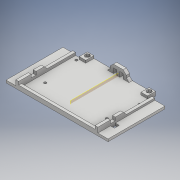
# Autodesk Inventor part: odroid_router
Saved by Autodesk Inventor 2018 (Build 220112000, 112)
## iProperties
Created: 2018-05-15
Part Number: odroid_router
Material: Generic
Document SubType Name: Modeling
Designer: bitbots
Density: 1 g/cm^3
Appearance: Default
Author: bitbots
Autodesk Inventor part; units mm, degrees
ref_plane "YZ Plane" through (0, 0, 0) normal (1, 0, 0) x (0, 1, 0)
ref_plane "XZ Plane" through (0, 0, 0) normal (0, 1, 0) x (-1, 0, 0)
ref_plane "Work Plane1" through (0, 0, 2) normal (0, 0, 1) x (1, 0, 0)
sketch "Sketch1" plane through (0, 0, 2) normal (0, 0, 1) x (1, 0, 0)
  arc A0 (0, 3.5) -> (-3.5, 0) centre (0, 0) ccw construction
  line L0 (-3.5, -52) -> (-3.5, 0) construction
  arc A1 (-3.5, -52) -> (0, -55.5) centre (0, -52) ccw construction
  line L1 (76, -55.5) -> (0, -55.5) construction
  arc A2 (76, -55.5) -> (79.5, -52) centre (76, -52) ccw construction
  line L2 (79.5, 0) -> (79.5, -52) construction
  arc A3 (79.5, 0) -> (76, 3.5) centre (76, 0) ccw construction
  line L3 (0, 3.5) -> (76, 3.5) construction
  circle A4 centre (0, -52) radius 1.4224 construction
  circle A5 centre (0, 0) radius 1.4224 construction
  circle A6 centre (76, 0) radius 1.4224 construction
  circle A7 centre (76, -52) radius 1.4224 construction
  circle A8 centre (25.43, -38.5) radius 1.4224 construction
  circle A9 centre (76.11, -18.5) radius 1.4224 construction
  circle A10 centre (76, 0) radius 1.5
  circle A11 centre (76, -52) radius 1.5
  circle A12 centre (76, -52) radius 3.5
  circle A13 centre (76, 0) radius 3.5
  circle A14 centre (0, -52) radius 1.5
  circle A15 centre (0, -52) radius 3.5
  circle A16 centre (0, 0) radius 1.5
  circle A17 centre (0, 0) radius 3.5
  dimension "d0" = 3
  dimension "d1" = 3
  dimension "d2" = 7
  dimension "d3" = 7
  dimension "d4" = 3
  dimension "d5" = 7
  dimension "d6" = 3
  dimension "d7" = 7
  constraints: 8 centre point, 8 coincident
  measures "d0" diameter of A10
  measures "d1" diameter of A11
  measures "d2" diameter of A12
  measures "d3" diameter of A13
  measures "d4" diameter of A14
  measures "d5" diameter of A15
  measures "d6" diameter of A16
  measures "d7" diameter of A17
extrude "Extrusion1" add sketch "Sketch1" against normal blind 4.5
sketch "Sketch2" plane through (0, 0, 2) normal (0, 0, 1) x (1, 0, 0)
  circle A0 centre (76, -52) radius 1.5 projected
  circle A1 centre (76, -52) radius 3.5 projected
  circle A2 centre (0, -52) radius 3.5 projected
  circle A3 centre (0, 0) radius 1.5 projected
  circle A4 centre (0, 0) radius 3.5 projected
  circle A5 centre (76, 0) radius 1.5 projected
  circle A6 centre (76, 0) radius 3.5 projected
  circle A7 centre (76, -52) radius 1.5 projected
  line L0 (76, -52) -> (76, -56)
  circle A8 centre (76, -52) radius 3.5 projected
  circle A9 centre (0, 0) radius 3.5 projected
  line L1 (0, 0) -> (-4, 0)
  circle A10 centre (0, -52) radius 1.5 projected
  circle A11 centre (0, -52) radius 3.5 projected
  line L2 (76, -56) -> (80, -56)
  line L3 (-4, 0) -> (-4, 4)
  line L4 (-4, 4) -> (80, 4)
  line L5 (80, 4) -> (80, -56)
  line L6 (80, -56) -> (-4, -56)
  line L7 (-4, -56) -> (-4, 4)
  point P0 (0, 0)
  dimension "d10" = 4
  dimension "d12" = 4
  dimension "d21" = 4
  dimension "d22" = 4
  constraints: 16 end point, 3 horizontal, 2 parallel, 2 vertical, 1 perpendicular, 1 vertical alignment
  measures "d10" distance of L0.start L0.end
  measures "d12" distance of L1.start L1.end
  measures "d21" distance of L0.end L2.end
  measures "d22" distance of L1.end L3.end
extrude "Extrusion2" add sketch "Sketch2" along normal blind 2 contours A1 | A4 | L6 L7 L3 L4 L5 L2 | A2 | A6
sketch "Sketch3" plane through (0, 0, 4) normal (0, 0, 1) x (1, 0, 0)
  circle A0 centre (76, 0) radius 1.5 construction
  circle A1 centre (0, 0) radius 1.5 construction
  circle A2 centre (0, -52) radius 1.5 construction
  circle A3 centre (76, -52) radius 1.5 construction
  circle A4 centre (0, 0) radius 1.5 construction
  line L0 (0, 0) -> (2.6, 0) construction
  line L1 (2.6, -1.5011) -> (0, -3.0022)
  line L2 (0, -3.0022) -> (-2.6, -1.5011)
  line L3 (-2.6, -1.5011) -> (-2.6, 1.5011)
  line L4 (-2.6, 1.5011) -> (0, 3.0022)
  line L5 (0, 3.0022) -> (2.6, 1.5011)
  line L6 (2.6, 1.5011) -> (2.6, -1.5011)
  line L7 (3.3236, -3.218) -> (-3.3236, 3.218) construction
  line L8 (-3.3236, -3.218) -> (3.3236, 3.218) construction
  line L9 (80, 4) -> (-4, 4) projected
  line L10 (-4, 4) -> (-4, -56) projected
  line L11 (4, -4) -> (-4, -4)
  line L12 (-4, -4) -> (-4, 4)
  line L13 (-4, 4) -> (4, 4)
  line L14 (4, 4) -> (4, -4)
  circle A5 centre (0, 0) radius 1.5 projected
  line L15 (4, -4) -> (-4, 4) construction
  line L16 (-4, -4) -> (4, 4) construction
  point P0 (0, 0)
  dimension "d18" = 2.6
  constraints: 30 end point, 5 midpoint, 2 horizontal, 2 parallel, 1 coincident, 1 perpendicular, 13 other
  measures "d18" distance of L0.start L0.end
extrude "Extrusion3" add sketch "Sketch3" along normal blind 3 contours L14 L11 L10 L9
ref_plane "Work Plane2" through (38, -56, 2) normal (1, 0, 0) x (0, 0, -1)
mirror "Mirror1" about plane through (38, -56, 2) normal (1, 0, 0) of "Extrusion3"
sketch "Sketch4" plane through (0, 0, 4) normal (0, 0, 1) x (1, 0, 0)
  circle A0 centre (76, -52) radius 1.5 projected
  circle A1 centre (0, -52) radius 1.5 projected
  line L0 (80, -4) -> (72, -4) projected
  line L1 (72, -4) -> (72, 4) projected
  line L2 (72, 4) -> (4, 4) projected
  line L3 (4, 4) -> (4, -4) projected
  line L4 (4, -4) -> (-4, -4) projected
  line L5 (-4, -4) -> (-4, -56) projected
  line L6 (-4, -56) -> (80, -56) projected
  line L7 (80, -56) -> (80, -4) projected
  line L8 (-4, 4) -> (-4, -56) projected
  line L9 (-4, -56) -> (-4, 4)
  line L10 (-4, -26) -> (38, -26)
  line L11 (-11, -48) -> (87, -48)
  line L12 (87, -48) -> (87, -4)
  line L13 (87, -4) -> (-11, -4)
  line L14 (-11, -4) -> (-11, -48)
  line L15 (-11, -48) -> (87, -4) construction
  line L16 (87, -48) -> (-11, -4) construction
  point P0 (0, 0)
  dimension "d23" = 98
  dimension "d24" = 44
  constraints: 16 end point, 3 midpoint, 2 horizontal, 2 parallel, 1 perpendicular, 1 vertical
  measures "d23" distance of L13.end L12.end
  measures "d24" distance of L11.end L12.end
extrude "Extrusion4" add sketch "Sketch4" against normal blind 2 contours L7 L11 L5 L4 L13 L0 | L13 L12 L11 L7 | L11 L14 L13 L5
sketch "Sketch5" plane through (0, 0, 4) normal (0, 0, 1) x (1, 0, 0)
  circle A0 centre (76, 0) radius 1.5 projected
  line L0 (76, 0) -> (76, -20)
  line L1 (76, -20) -> (81, -20)
  circle A1 centre (81, -20) radius 1.5
  circle A2 centre (0, 0) radius 1.5 projected
  line L2 (0, 0) -> (0, -12)
  line L3 (0, -12) -> (-5, -12)
  circle A3 centre (-5, -12) radius 1.5
  point P0 (0, 0)
  dimension "d27" = 20
  dimension "d28" = 5
  dimension "d29" = 3
  dimension "d30" = 12
  dimension "d31" = 5
  dimension "d32" = 3
  constraints: 8 end point, 2 centre point, 2 coincident, 2 vertical, 1 horizontal, 1 perpendicular
  measures "d27" distance of L0.start L0.end
  measures "d28" distance of L0.end L1.end
  measures "d29" diameter of A1
  measures "d30" distance of L2.start L2.end
  measures "d31" distance of L2.end L3.end
  measures "d32" diameter of A3
extrude "Extrusion5" cut sketch "Sketch5" against normal blind 2 contours A1 | A3
sketch "Sketch7" plane through (-11, -48, 4) normal (-1, 0, 0) x (0, 0, 1)
  line L0 (0, 44) -> (0, 0) projected
  line L1 (0, 44) -> (-2, 44) projected
  line L2 (-2, 0) -> (-2, 44) projected
  line L3 (0, 0) -> (-2, 0) projected
  point P0 (-4, 48)
extrude "Extrusion6" add sketch "Sketch7" along normal blind 3
sketch "Sketch6" plane through (0, 0, 4) normal (0, 0, 1) x (1, 0, 0)
  circle A0 centre (81, -20) radius 1.5 projected
  circle A1 centre (-5, -12) radius 1.5 projected
  circle A2 centre (0, -52) radius 1.5 projected
  circle A3 centre (76, -52) radius 1.5 projected
  line L0 (72, -4) -> (72, 4) projected
  line L1 (72, 4) -> (4, 4) projected
  line L2 (4, 4) -> (4, -4) projected
  line L3 (4, -4) -> (-4, -4) projected
  line L4 (-4, -4) -> (-14, -4) projected
  line L5 (-14, -48) -> (-4, -48) projected
  line L6 (-4, -48) -> (-4, -56) projected
  line L7 (-4, -56) -> (80, -56) projected
  line L8 (80, -56) -> (80, -48) projected
  line L9 (80, -48) -> (87, -48) projected
  line L10 (87, -48) -> (87, -4) projected
  line L11 (87, -4) -> (80, -4) projected
  line L12 (80, -4) -> (72, -4) projected
  line L13 (81, -20) -> (83.5, -20)
  line L14 (83.5, -20) -> (83.5, -4)
  line L15 (80, -4) -> (87, -4) projected
  line L16 (87, -4) -> (83.5, -4)
  line L17 (87, -48) -> (87, -4) projected
  line L18 (87, -4) -> (87, -48)
  line L19 (83.5, -20) -> (83.5, -48)
  line L20 (80, -48) -> (87, -48) projected
  line L21 (87, -48) -> (83.5, -48)
  circle A4 centre (-5, -12) radius 1.5 projected
  line L22 (-5, -12) -> (-10.5, -12)
  line L23 (-14, -48) -> (-14, -4) projected
  line L24 (-10.5, -12) -> (-10.5, -4)
  line L25 (-4, -4) -> (-14, -4) projected
  line L26 (-14, -4) -> (-10.5, -4)
  line L27 (-4, -48) -> (-14, -48) projected
  line L28 (-14, -4) -> (-14, -48)
  line L29 (-14, -48) -> (-10.5, -48)
  line L30 (-10.5, -48) -> (-10.5, -12)
  point P0 (0, 0)
  dimension "d35" = 2.5
  dimension "d36" = 5.5
  constraints: 24 end point, 5 collinear, 3 point on line, 2 horizontal, 2 midpoint, 2 vertical
  measures "d35" distance of L13.start L13.end
  measures "d36" distance of L22.start L22.end
extrude "Extrusion7" add sketch "Sketch6" along normal blind 3.3 contours L14 L11 L10 L9 L19 | L5 L23 L4 L24 L30
sketch "Sketch8" plane through (0, 0, 4) normal (0, 0, 1) x (1, 0, 0)
  line L0 (83.5, -48) -> (83.5, -4) projected
  line L1 (83.5, -4) -> (80, -4) projected
  line L2 (80, -4) -> (72, -4) projected
  line L3 (72, -4) -> (72, 4) projected
  line L4 (72, 4) -> (4, 4) projected
  line L5 (4, 4) -> (4, -4) projected
  line L6 (4, -4) -> (-4, -4) projected
  line L7 (-4, -4) -> (-10.5, -4) projected
  line L8 (-10.5, -4) -> (-10.5, -48) projected
  line L9 (-10.5, -48) -> (-4, -48) projected
  line L10 (-4, -48) -> (-4, -56) projected
  line L11 (-4, -56) -> (80, -56) projected
  line L12 (80, -56) -> (80, -48) projected
  line L13 (80, -48) -> (83.5, -48) projected
  circle A0 centre (81, -20) radius 1.5 projected
  circle A1 centre (-5, -12) radius 1.5 projected
  circle A2 centre (0, -52) radius 1.5 projected
  circle A3 centre (76, -52) radius 1.5 projected
  circle A4 centre (81, -20) radius 1.5 projected
  line L14 (81, -20) -> (81, -74)
  line L15 (-14, -4) -> (-14, -48) projected
  line L16 (-14, -48) -> (-10.5, -48) projected
  line L17 (-10.5, -48) -> (-10.5, -4) projected
  line L18 (-10.5, -4) -> (-14, -4) projected
  line L19 (87, -48) -> (87, -4) projected
  line L20 (87, -4) -> (83.5, -4) projected
  line L21 (83.5, -4) -> (83.5, -48) projected
  line L22 (83.5, -48) -> (87, -48) projected
  line L23 (81, -74) -> (87, -74)
  line L24 (80, -48) -> (87, -48)
  line L25 (87, -48) -> (87, -74)
  line L26 (87, -74) -> (80, -74)
  line L27 (80, -74) -> (80, -48)
  line L28 (-10.5, -48) -> (-4, -48)
  line L29 (-4, -48) -> (-4, -74)
  line L30 (-4, -74) -> (-10.5, -74)
  line L31 (-10.5, -74) -> (-10.5, -48)
  line L32 (-4, -74) -> (80, -74)
  line L33 (80, -74) -> (80, -56)
  line L34 (80, -56) -> (-4, -56)
  line L35 (-4, -56) -> (-4, -74)
  line L36 (-4, -48) -> (-14, -48) projected
  line L37 (-14, -48) -> (-10.5, -48)
  line L38 (-10.5, -48) -> (-10.5, -74)
  line L39 (-10.5, -74) -> (-14, -74)
  line L40 (-14, -74) -> (-14, -48)
  point P0 (0, 0)
  dimension "d41" = 54
  constraints: 36 end point, 8 parallel, 5 horizontal, 4 perpendicular, 1 point on line, 1 vertical
  measures "d41" distance of L14.start L14.end
extrude "Extrusion8" add sketch "Sketch8" against normal blind 2 contours L22 L25 L23 L14 L13 | L14 L26 L27 L12 L13 | L27 L32 L29 L11 | L29 L30 L31 L9 L10 | L39 L40 L16 L31 | L16 L15 L18 L8
sketch "Sketch9" plane through (0, 0, 4) normal (0, 0, 1) x (1, 0, 0)
  line L0 (83.5, -48) -> (83.5, -4) projected
  line L1 (83.5, -4) -> (80, -4) construction
  line L2 (80, -4) -> (72, -4) construction
  line L3 (72, -4) -> (72, 4) construction
  line L4 (72, 4) -> (4, 4) construction
  line L5 (4, 4) -> (4, -4) construction
  line L6 (4, -4) -> (-4, -4) construction
  line L7 (-4, -4) -> (-10.5, -4) projected
  line L8 (-10.5, -4) -> (-10.5, -48) projected
  line L9 (-14, -48) -> (-10.5, -48) projected
  line L10 (-14, -48) -> (-14, -74) projected
  line L11 (-14, -74) -> (87, -74) projected
  line L12 (87, -74) -> (87, -48) projected
  line L13 (83.5, -48) -> (87, -48) projected
  circle A0 centre (81, -20) radius 1.5 construction
  circle A1 centre (-5, -12) radius 1.5 projected
  circle A2 centre (0, -52) radius 1.5 projected
  circle A3 centre (76, -52) radius 1.5 projected
  line L14 (-14, -74) -> (87, -74) projected
  line L15 (-14, -48) -> (-10.5, -48)
  line L16 (-10.5, -48) -> (-10.5, -74)
  line L17 (-10.5, -74) -> (-14, -74)
  line L18 (-14, -74) -> (-14, -48)
  line L19 (87, -48) -> (87, -4) projected
  line L20 (87, -48) -> (83.5, -48)
  line L21 (83.5, -48) -> (83.5, -74)
  line L22 (83.5, -74) -> (87, -74)
  line L23 (87, -74) -> (87, -48)
  line L24 (83.5, -74) -> (-10.5, -74)
  line L25 (-10.5, -74) -> (-10.5, -70.7)
  line L26 (-10.5, -70.7) -> (83.5, -70.7)
  line L27 (83.5, -70.7) -> (83.5, -74)
  point P0 (0, 0)
  dimension "d44" = 3.3
  constraints: 24 end point, 6 parallel, 3 horizontal, 3 perpendicular, 3 point on line
  measures "d44" distance of L24.end L25.end
extrude "Extrusion9" add sketch "Sketch9" along normal up to surface (3.3 mm away) contours L9 L16 L11 L10 | L26 L21 L11 L16 | L21 L13 L12 L11
sketch "Sketch10" plane through (-14, -48, 4) normal (-1, 0, 0) x (0, 0, 1)
  line L0 (-6.5, 51.5) -> (-6.5, 44.5) projected
  line L1 (-2, 51.5) -> (-2, 44.5) projected
  line L2 (-6.5, -0.5) -> (-6.5, -7.5) projected
  line L3 (-2, -0.5) -> (-2, -7.5) projected
  line L4 (-6.5, 51.5) -> (-6.5, 44.5) projected
  line L5 (-6.5, 51.5) -> (-2, 51.5)
  line L6 (-2, 51.5) -> (-2, 44.5)
  line L7 (-2, 44.5) -> (-6.5, 44.5)
  line L8 (-6.5, 44.5) -> (-6.5, 51.5)
  line L9 (-2, -0.5) -> (-6.5, -0.5)
  line L10 (-6.5, -0.5) -> (-6.5, -7.5)
  line L11 (-6.5, -7.5) -> (-2, -7.5)
  line L12 (-2, -7.5) -> (-2, -0.5)
  point P0 (-4, 48)
  constraints: 16 end point, 4 parallel, 2 horizontal, 2 perpendicular
extrude "Extrusion10" cut sketch "Sketch10" against normal through all
sketch "Sketch11" plane through (0, 0, 7.3) normal (0, 0, 1) x (1, 0, 0)
  line L0 (-14, -4) -> (-14, -74) projected
  line L1 (87, -74) -> (-14, -74) projected
  line L2 (87, -4) -> (87, -74) projected
  line L3 (87, -4) -> (83.5, -4) projected
  line L4 (83.5, -4) -> (83.5, -70.7) projected
  line L5 (-10.5, -70.7) -> (83.5, -70.7) projected
  line L6 (-10.5, -4) -> (-10.5, -70.7) projected
  line L7 (-10.5, -4) -> (-14, -4) projected
  line L8 (-10.5, -70.7) -> (-10.5, -58.7)
  line L9 (-10.5, -4) -> (-10.5, -70.7) projected
  line L10 (-10.5, -70.7) -> (-10.5, -52.7)
  line L11 (-14, -4) -> (-14, -74) projected
  line L12 (-10.5, -52.7) -> (-14, -52.7)
  line L13 (-14, -52.7) -> (-14, -42.7)
  line L14 (-14, -42.7) -> (-10.5, -42.7)
  line L15 (-10.5, -42.7) -> (-10.5, -52.7)
  line L16 (-10.5, -58.7) -> (-14, -58.7)
  line L17 (-14, -58.7) -> (-14, -74)
  line L18 (-14, -74) -> (-10.5, -74)
  line L19 (-10.5, -74) -> (-10.5, -58.7)
  line L20 (87, -4) -> (87, -74) projected
  line L21 (83.5, -42.7) -> (87, -42.7)
  line L22 (87, -42.7) -> (87, -52.7)
  line L23 (87, -52.7) -> (83.5, -52.7)
  line L24 (83.5, -52.7) -> (83.5, -42.7)
  line L25 (83.5, -70.7) -> (83.5, -4) projected
  line L26 (83.5, -58.7) -> (87, -58.7)
  line L27 (87, -58.7) -> (87, -74)
  line L28 (87, -74) -> (83.5, -74)
  line L29 (83.5, -74) -> (83.5, -58.7)
  point P0 (0, 0)
  dimension "d49" = 12
  dimension "d50" = 18
  dimension "d51" = 10
  constraints: 36 end point, 8 parallel, 6 point on line, 4 horizontal, 4 perpendicular
  measures "d49" distance of L5.start L8.end
  measures "d50" distance of L5.start L10.end
  measures "d51" distance of L12.end L13.end
extrude "Extrusion11" add sketch "Sketch11" along normal blind 4 contours L14 L6 L12 L0 | L16 L6 L19 L1 L0 | L29 L4 L26 L2 L1 | L4 L21 L2 L23
chamfer "Chamfer1" distance 4 angle 45 2 edges at (85.25, -42.7, 7.3) (-12.25, -42.7, 7.3)
sketch "Sketch12" plane through (0, 0, 7.3) normal (0, 0, 1) x (1, 0, 0)
  line L0 (87, -38.7) -> (83.5, -38.7) projected
  line L1 (87, -4) -> (87, -38.7) projected
  line L2 (87, -4) -> (83.5, -4) projected
  line L3 (83.5, -4) -> (83.5, -38.7) projected
  circle A0 centre (76, -52) radius 1.5 projected
  circle A1 centre (0, -52) radius 1.5 projected
  circle A2 centre (-5, -12) radius 1.5 projected
  circle A3 centre (81, -20) radius 1.5 projected
  line L4 (-10.5, -4) -> (-10.5, -70.7) projected
  line L5 (-10.5, -70.7) -> (83.5, -70.7) projected
  line L6 (83.5, -70.7) -> (83.5, -4) projected
  line L7 (83.5, -4) -> (80, -4) projected
  line L8 (80, -4) -> (72, -4) projected
  line L9 (72, -4) -> (72, 4) projected
  line L10 (72, 4) -> (4, 4) projected
  line L11 (4, 4) -> (4, -4) projected
  line L12 (4, -4) -> (-4, -4) projected
  line L13 (-4, -4) -> (-10.5, -4) projected
  line L14 (87, -4) -> (80, -4)
  line L15 (80, -4) -> (80, -15)
  line L16 (80, -15) -> (87, -15)
  line L17 (87, -15) -> (87, -4)
  point P0 (0, 0)
  dimension "d57" = 7
  dimension "d58" = 11
  constraints: 8 end point, 2 parallel, 1 horizontal, 1 perpendicular
  measures "d57" distance of L16.end L15.end
  measures "d58" distance of L15.end L14.end
extrude "Extrusion12" cut sketch "Sketch12" against normal through all contours L16 L3 L2 L1 | L16 L15 L7 L3
sketch "Sketch13" plane through (0, 0, 2) normal (0, 0, -1) x (-1, 0, 0)
  circle A0 centre (-81, -20) radius 1.5 projected
  circle A1 centre (5, -12) radius 1.5 projected
  line L0 (-80, -15) -> (-80, 4) projected
  line L1 (-80, -15) -> (-87, -15) projected
  line L2 (-87, -15) -> (-87, -74) projected
  line L3 (-87, -74) -> (14, -74) projected
  line L4 (14, -4) -> (14, -74) projected
  line L5 (4, -4) -> (14, -4) projected
  line L6 (4, 4) -> (4, -4) projected
  line L7 (-80, 4) -> (4, 4) projected
  circle A2 centre (0, -52) radius 1.5 projected
  circle A3 centre (-76, -52) radius 1.5 projected
  circle A4 centre (-76, 0) radius 1.5 projected
  circle A5 centre (0, 0) radius 1.5 projected
  line L8 (14, -74) -> (24, -74)
  line L9 (24, -74) -> (24, -4)
  line L10 (24, -4) -> (14, -4)
  line L11 (14, -4) -> (14, -74)
  line L12 (-87, -74) -> (-97, -74)
  line L13 (-97, -74) -> (-97, -15)
  line L14 (-97, -15) -> (-87, -15)
  line L15 (-87, -15) -> (-87, -74)
  point P0 (0, 0)
  dimension "d61" = 10
  dimension "d62" = 10
  constraints: 16 end point, 4 parallel, 2 horizontal, 2 perpendicular
  measures "d61" distance of L10.end L9.end
  measures "d62" distance of L13.end L14.end
extrude "Extrusion13" add sketch "Sketch13" against normal blind 3 contours L2 L12 L13 L14 | L4 L10 L9 L8
sketch "Sketch14" plane through (0, 0, 2) normal (0, 0, -1) x (-1, 0, 0)
  line L0 (14, -58.7) -> (10.5, -58.7) projected
  line L1 (10.5, -52.7) -> (10.5, -58.7) projected
  line L2 (10.5, -52.7) -> (14, -52.7) projected
  line L3 (14, -52.7) -> (14, -58.7) projected
  line L4 (-83.5, -58.7) -> (-87, -58.7) projected
  line L5 (-87, -52.7) -> (-87, -58.7) projected
  line L6 (-87, -52.7) -> (-83.5, -52.7) projected
  line L7 (-83.5, -52.7) -> (-83.5, -58.7) projected
  line L8 (14, -58.7) -> (14, -74) projected
  line L9 (14, -58.7) -> (19, -58.7)
  line L10 (19, -58.7) -> (19, -52.7)
  line L11 (19, -52.7) -> (14, -52.7)
  line L12 (14, -52.7) -> (14, -58.7)
  line L13 (-87, -58.7) -> (-83.5, -58.7) projected
  line L14 (-87, -58.7) -> (-92, -58.7)
  line L15 (-92, -58.7) -> (-92, -52.7)
  line L16 (-92, -52.7) -> (-87, -52.7)
  line L17 (-87, -52.7) -> (-87, -58.7)
  point P0 (0, 0)
  dimension "d65" = 5
  dimension "d66" = 5
  constraints: 16 end point, 4 parallel, 2 horizontal, 2 perpendicular, 1 point on line
  measures "d65" distance of L11.end L10.end
  measures "d66" distance of L15.end L16.end
extrude "Extrusion14" cut sketch "Sketch14" against normal through all contours L3 L11 L10 L9 | L14 L15 L16 L5
sketch "Sketch15" plane through (-10.5, -74, 7.3) normal (0, -1, 0) x (1, 0, 0)
  line L0 (107.5, -5.3) -> (-13.5, -5.3) projected
  line L1 (107.5, -5.3) -> (107.5, -2.3) projected
  line L2 (97.5, -2.3) -> (107.5, -2.3) projected
  line L3 (97.5, -2.3) -> (97.5, 4) projected
  line L4 (94, 4) -> (97.5, 4) projected
  line L5 (94, 0) -> (94, 4) projected
  line L6 (94, 0) -> (0, 0) projected
  line L7 (0, 0) -> (0, 4) projected
  line L8 (-3.5, 4) -> (0, 4) projected
  line L9 (-3.5, -2.3) -> (-3.5, 4) projected
  line L10 (-13.5, -2.3) -> (-3.5, -2.3) projected
  line L11 (-13.5, -5.3) -> (-13.5, -2.3) projected
  line L12 (107.5, -5.3) -> (109.5, -5.3)
  line L13 (109.5, -5.3) -> (109.5, -2.3)
  line L14 (109.5, -2.3) -> (107.5, -2.3)
  line L15 (107.5, -2.3) -> (107.5, -5.3)
  point P0 (10.5, -7.3)
  dimension "d69" = 2
  constraints: 8 end point, 2 parallel, 1 horizontal, 1 perpendicular
  measures "d69" distance of L14.end L13.end
extrude "Extrusion15" add sketch "Sketch15" against normal up to surface (59 mm away) contours L1 L14 L13 L12
sketch "Sketch16" plane through (-24, -74, 2) normal (-1, 0, 0) x (0, 0, 1)
  line L0 (0, 0) -> (0, 70) projected
  line L1 (0, 0) -> (3, 0) projected
  line L2 (3, 70) -> (3, 0) projected
  line L3 (0, 70) -> (3, 70) projected
  point P0 (-2, 74)
extrude "Extrusion16" add sketch "Sketch16" along normal blind 3
sketch "Sketch17" plane through (0, 0, 4) normal (0, 0, 1) x (1, 0, 0)
  line L0 (80, -15) -> (80, -4) projected
  line L1 (80, -4) -> (72, -4) projected
  line L2 (72, -4) -> (72, 4) projected
  line L3 (72, 4) -> (4, 4) projected
  line L4 (4, 4) -> (4, -4) projected
  line L5 (4, -4) -> (-4, -4) projected
  line L6 (-4, -4) -> (-10.5, -4) projected
  line L7 (-10.5, -4) -> (-10.5, -70.7) projected
  line L8 (-10.5, -70.7) -> (83.5, -70.7) projected
  line L9 (83.5, -70.7) -> (83.5, -15) projected
  line L10 (83.5, -15) -> (80, -15) projected
  circle A0 centre (76, -52) radius 1.5 projected
  circle A1 centre (0, -52) radius 1.5 projected
  circle A2 centre (-5, -12) radius 1.5 projected
  circle A3 centre (81, -20) radius 1.5 projected
  line L11 (80, 4) -> (-4, 4) projected
  line L12 (38, 4) -> (36, 4)
  line L13 (36, 4) -> (36, 0)
  line L14 (36, 0) -> (38, 0)
  line L15 (38, 0) -> (38, 4)
  line L16 (38, 0) -> (40, 0)
  line L17 (40, 0) -> (40, 4)
  line L18 (40, 4) -> (38, 4)
  line L19 (38, 4) -> (38, 0)
  line L20 (40, 0) -> (44, 0)
  line L21 (36, 0) -> (32, 0)
  line L22 (44, 0) -> (48, 0)
  line L23 (48, 0) -> (48, 4)
  line L24 (48, 4) -> (44, 4)
  line L25 (44, 4) -> (44, 0)
  line L26 (32, 0) -> (28, 0)
  line L27 (28, 0) -> (28, 4)
  line L28 (28, 4) -> (32, 4)
  line L29 (32, 4) -> (32, 0)
  point P0 (0, 0)
  dimension "d74" = 2
  dimension "d75" = 4
  dimension "d76" = 2
  dimension "d77" = 4
  dimension "d78" = 4
  dimension "d79" = 4
  dimension "d80" = 4
  dimension "d81" = 4
  dimension "d82" = 4
  dimension "d83" = 4
  constraints: 36 end point, 8 parallel, 6 horizontal, 4 perpendicular, 1 midpoint
  measures "d74" distance of L14.end L13.end
  measures "d75" distance of L13.end L12.end
  measures "d76" distance of L18.end L17.end
  measures "d77" distance of L17.end L16.end
  measures "d78" distance of L16.end L20.end
  measures "d79" distance of L13.end L21.end
  measures "d80" distance of L24.end L23.end
  measures "d81" distance of L23.end L22.end
  measures "d82" distance of L27.end L28.end
  measures "d83" distance of L26.end L27.end
extrude "Extrusion17" add sketch "Sketch17" along normal blind 6 contours L23 L22 L25 L3 | L17 L16 L15 L3 | L15 L14 L13 L3 | L3 L29 L26 L27
sketch "Sketch18" plane through (0, 0, 10) normal (0, 0, 1) x (1, 0, 0)
  line L0 (32, 0) -> (32, 4) projected
  line L1 (32, 4) -> (28, 4) projected
  line L2 (28, 4) -> (28, 0) projected
  line L3 (28, 0) -> (32, 0) projected
  line L4 (40, 4) -> (36, 4) projected
  line L5 (36, 4) -> (36, 0) projected
  line L6 (36, 0) -> (40, 0) projected
  line L7 (40, 0) -> (40, 4) projected
  line L8 (44, 0) -> (48, 0) projected
  line L9 (48, 0) -> (48, 4) projected
  line L10 (48, 4) -> (44, 4) projected
  line L11 (44, 4) -> (44, 0) projected
  line L12 (48, 4) -> (44, 4) projected
  line L13 (28, 0) -> (48, 0)
  line L14 (48, 0) -> (48, 4)
  line L15 (48, 4) -> (28, 4)
  line L16 (28, 4) -> (28, 0)
  point P0 (0, 0)
  constraints: 8 end point, 2 parallel, 1 horizontal, 1 perpendicular
extrude "Extrusion18" add sketch "Sketch18" along normal blind 4
chamfer "Chamfer2" distance 3.3 angle 45 2 edges at (48, 2, 4) (28, 2, 4)
chamfer "Chamfer3" distance 4 angle 45 2 edges at (48, 2, 14) (28, 2, 14)
sketch "Sketch19" plane through (-10.5, -70.7, 4) normal (0, 1, 0) x (1, 0, 0)
  line L0 (0, -3.3) -> (94, -3.3) projected
  line L1 (94, 0) -> (94, -3.3) projected
  line L2 (0, 0) -> (94, 0) projected
  line L3 (0, -3.3) -> (0, 0) projected
  point P0 (10.5, 4)
extrude "Extrusion19" add sketch "Sketch19" along normal blind 0.2
sketch "Sketch20" plane through (-4, -4, 7) normal (0, -1, 0) x (1, 0, 0)
  line L0 (2.5, -3) -> (5.5, -3) projected
  line L1 (8, -3) -> (0, -3) projected
  line L2 (8, -3) -> (8, 0) projected
  line L3 (0, 0) -> (8, 0) projected
  line L4 (0, -3) -> (0, 0) projected
  line L5 (84, -3) -> (76, -3) projected
  line L6 (84, -3) -> (84, 0) projected
  line L7 (84, 0) -> (76, 0) projected
  line L8 (76, -3) -> (76, 0) projected
  point P0 (4, -7)
extrude "Extrusion20" add sketch "Sketch20" along normal blind 2
sketch "Sketch21" plane through (0, 0, 2) normal (0, 0, -1) x (-1, 0, 0)
  line L0 (4, -4) -> (27, -4) projected
  line L1 (-80, -15) -> (-99, -15) projected
  line L2 (-99, -74) -> (-99, -15) projected
  line L3 (-99, -15) -> (-80, -15)
  line L4 (-80, -15) -> (-80, -4)
  line L5 (-80, -4) -> (-99, -4)
  line L6 (-99, -4) -> (-99, -15)
  point P0 (0, 0)
  constraints: 8 end point, 2 parallel, 1 horizontal, 1 perpendicular
extrude "Extrusion21" add sketch "Sketch21" against normal up to surface (2 mm away)
sketch "Sketch22" plane through (83.5, -15, 7.3) normal (0, 1, 0) x (1, 0, 0)
  line L0 (15.5, 3.3) -> (0, 3.3) projected
  line L1 (0, 0) -> (0, 3.3) projected
  line L2 (3.5, 0) -> (0, 0) projected
  line L3 (3.5, 2.3) -> (3.5, 0) projected
  line L4 (3.5, 2.3) -> (15.5, 2.3) projected
  line L5 (15.5, 2.3) -> (15.5, 3.3) projected
  line L6 (0, 0) -> (0, -4) projected
  line L7 (3.5, -4) -> (0, -4) projected
  line L8 (3.5, -4) -> (3.5, 0) projected
  line L9 (3.5, 0) -> (0, 0) projected
  point P0 (-83.5, 7.3)
extrude "Extrusion22" add sketch "Sketch22" along normal up to surface (11 mm away) contours L5 L4 L3 L2 L1 L0
sketch "Sketch23" plane through (0, 0, 4) normal (0, 0, 1) x (1, 0, 0)
  line L0 (83.5, -70.5) -> (83.5, -4) projected
  line L1 (80, -4) -> (83.5, -4) projected
  line L2 (80, -6) -> (80, -4) projected
  line L3 (80, -6) -> (72, -6) projected
  line L4 (72, -6) -> (72, 4) projected
  line L5 (72, 4) -> (51.3, 4) projected
  line L6 (51.3, 0) -> (51.3, 4) projected
  line L7 (51.3, 0) -> (44, 0) projected
  line L8 (44, 0) -> (44, 4) projected
  line L9 (44, 4) -> (40, 4) projected
  line L10 (40, 4) -> (40, 0) projected
  line L11 (40, 0) -> (36, 0) projected
  line L12 (36, 0) -> (36, 4) projected
  line L13 (36, 4) -> (32, 4) projected
  line L14 (32, 4) -> (32, 0) projected
  line L15 (32, 0) -> (24.7, 0) projected
  line L16 (24.7, 4) -> (24.7, 0) projected
  line L17 (24.7, 4) -> (4, 4) projected
  line L18 (4, 4) -> (4, -6) projected
  line L19 (4, -6) -> (-4, -6) projected
  line L20 (-4, -6) -> (-4, -4) projected
  line L21 (-4, -4) -> (-10.5, -4) projected
  line L22 (-10.5, -4) -> (-10.5, -70.5) projected
  line L23 (-10.5, -70.5) -> (83.5, -70.5) projected
  circle A0 centre (76, -52) radius 1.5 projected
  circle A1 centre (0, -52) radius 1.5 projected
  circle A2 centre (-5, -12) radius 1.5 projected
  circle A3 centre (81, -20) radius 1.5 projected
  circle A4 centre (-5, -12) radius 1.5 projected
  line L24 (-5, -12) -> (-5, -8.5)
  circle A5 centre (81, -20) radius 1.5 projected
  line L25 (81, -20) -> (81, -16.5)
  circle A6 centre (-5, -8.5) radius 1.5
  circle A7 centre (81, -16.5) radius 1.5
  point P0 (0, 0)
  dimension "d102" = 3.5
  dimension "d103" = 3.5
  dimension "d104" = 3
  dimension "d105" = 3
  constraints: 4 end point, 2 centre point, 2 coincident, 2 vertical
  measures "d102" distance of L24.start L24.end
  measures "d103" distance of L25.start L25.end
  measures "d104" diameter of A6
  measures "d105" diameter of A7
extrude "Extrusion23" cut sketch "Sketch23" against normal through all contours A6 | A7
sketch "Sketch24" plane through (0, 0, 4) normal (0, 0, 1) x (1, 0, 0)
  circle A0 centre (-5, -12) radius 1.5 projected
  circle A1 centre (81, -20) radius 1.5 projected
  point P0 (0, 0)
extrude "Extrusion24" add sketch "Sketch24" against normal up to surface (2 mm away)
sketch "Sketch25" plane through (-27, -74, 2) normal (-1, 0, 0) x (0, 0, 1)
  line L0 (0, 70) -> (0, 0) projected
  line L1 (0, 0) -> (3, 0) projected
  line L2 (3, 0) -> (3, 70) projected
  line L3 (3, 70) -> (0, 70) projected
  point P0 (-2, 74)
extrude "Extrusion25" cut sketch "Sketch25" against normal blind 1
sketch "Sketch26" plane through (99, -74, 5) normal (1, 0, 0) x (0, 0, -1)
  line L0 (0, 0) -> (0, 70) projected
  line L1 (3, 0) -> (0, 0) projected
  line L2 (3, 70) -> (3, 0) projected
  line L3 (3, 70) -> (0, 70) projected
  point P0 (5, 74)
extrude "Extrusion26" add sketch "Sketch26" along normal blind 0.5
body "Solid1"
